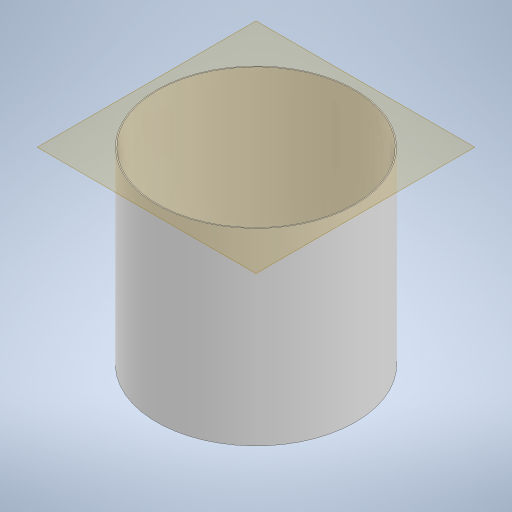
# Autodesk Inventor part: ejercicio1
Saved by Autodesk Inventor 2023.2 (Build 272271030, 271C)
## iProperties
Created: 2023-07-10
Part Number: ejercicio1
Material: Generic
Document SubType Name: Modeling
Designer: Cris Pat
Density: 1 g/cm^3
Appearance: Default
Author: Cris Pat
Autodesk Inventor part; units mm, degrees
ref_plane "YZ Plane" through (0, 0, 0) normal (1, 0, 0) x (0, 1, 0)
ref_plane "XZ Plane" through (0, 0, 0) normal (0, 1, 0) x (-1, 0, 0)
ref_plane "XY Plane" through (0, 0, 0) normal (0, 0, 1) x (1, 0, 0)
sketch "Sketch1" plane through (0, 0, 0) normal (0, 1, 0) x (-1, 0, 0)
  circle A0 centre (0, 0) radius 950
  dimension "d0" = 1900
  constraints: 1 centre point, 1 coincident
  measures "d0" diameter of A0
extrude "Extrusion1" add sketch "Sketch1" along normal blind 1800
ref_plane "Work Plane1" through (0, 1800, 0) normal (0, 1, 0) x (1, 0, 0)
sketch "Sketch2" plane through (0, 1800, 0) normal (0, 1, 0) x (1, 0, 0)
  circle A0 centre (0, 0) radius 950 construction
  circle A1 centre (0, 0) radius 940.475
  dimension "d4" = 9.525
  constraints: 1 centre point
  measures "d4" radial gap between concentric circles of A0 A1
extrude "Extrusion2" cut sketch "Sketch2" against normal blind 1800
body "Solid1"
